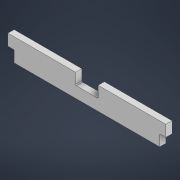
# Autodesk Inventor part: Breadth Board
Saved by Autodesk Inventor 2021 (Build 250183000, 183)
## iProperties
Created: 2021-03-26
Part Number: Breadth Board
Material: Generic
Document SubType Name: Modeling
Designer: allen
Density: 1 g/cm^3
Appearance: Default
Author: allen
Autodesk Inventor part; units mm, degrees
ref_plane "YZ Plane" through (0, 0, 0) normal (1, 0, 0) x (0, 1, 0)
ref_plane "XZ Plane" through (0, 0, 0) normal (0, 1, 0) x (-1, 0, 0)
sketch "Sketch1" plane through (0, 0, 0) normal (0, 0, 1) x (1, 0, 0)
  line L0 (0, 0) -> (384, 0)
  line L1 (384, 0) -> (384, 55)
  line L2 (384, 55) -> (0, 55)
  line L3 (0, 55) -> (0, 0)
  dimension "d0" = 55
  dimension "d1" = 384
  constraints: 8 end point, 2 parallel, 1 horizontal, 1 perpendicular
  measures "d0" distance of L2.end L0.start
  measures "d1" distance of L0.start L0.end
extrude "Extrusion1" add sketch "Sketch1" along normal blind 15
sketch "Sketch4" plane through (0, 0, 15) normal (0, 0, 1) x (1, 0, 0)
  line L0 (0, 0) -> (15, 0)
  line L1 (15, 0) -> (15, 27.5)
  line L2 (15, 27.5) -> (0, 27.5)
  line L3 (0, 27.5) -> (0, 0)
  line L4 (384, 55) -> (0, 55) projected
  line L5 (192, 55) -> (192, 39.783)
  line L6 (164.5, 55) -> (219.5, 55)
  line L7 (219.5, 55) -> (219.5, 27.5)
  line L8 (219.5, 27.5) -> (164.5, 27.5)
  line L9 (164.5, 27.5) -> (164.5, 55)
  line L10 (384, 0) -> (369, 0)
  line L11 (369, 0) -> (369, 27.5)
  line L12 (369, 27.5) -> (384, 27.5)
  line L13 (384, 27.5) -> (384, 0)
  point P0 (192, 27.5)
  dimension "d23" = 15
  dimension "d24" = 27.5
  dimension "d25" = 55
  constraints: 26 end point, 4 parallel, 4 symmetric about line, 2 horizontal, 2 midpoint, 2 perpendicular, 1 collinear, 1 point on line, 1 vertical, 1 vertical alignment
  measures "d23" distance of L1.end L2.end
  measures "d24" distance of L0.end L1.end
  measures "d25" distance of L7.end L8.end
extrude "Extrusion2" cut sketch "Sketch4" against normal through all
ref_plane "Work Plane1" through (192, 55, 15) normal (1, 0, 0) x (0, 0, -1)
fillet "Fillet1" radius 2 4 edges at (15, 27.5, 7.5) (164.5, 27.5, 7.5) (219.5, 27.5, 7.5) (369, 27.5, 7.5)
sketch "Sketch2" plane through (0, 55, 0) normal (0, 1, 0) x (1, 0, 0)
  line L0 (7.5, -7.5) -> (376.5, -7.5)
  line L1 (0, 0) -> (0, -15) projected
  line L2 (384, 0) -> (0, 0) projected
  point P0 (192, -7.5)
  point P1 (0, -7.5)
  point P2 (192, 0)
  dimension "d4" = 369
  constraints: 3 midpoint, 2 end point, 2 horizontal alignment, 1 horizontal, 1 vertical alignment
  measures "d4" distance of L0.start L0.end
sketch "Sketch3" plane through (0, 0, 0) normal (0, 0, -1) x (-1, 0, 0)
  line L0 (-384, 0) -> (-384, 55) projected
  line L1 (0, 0) -> (-384, 0) projected
  line L2 (0, 55) -> (0, 0) projected
  line L3 (-384, 55) -> (0, 55) projected
  line L4 (-7.5, 10) -> (-376.5, 10)
  line L5 (-376.5, 45) -> (-7.5, 45)
  dimension "d12" = 10
  dimension "d20" = 10
  dimension "d21" = 7.5
  dimension "d22" = 7.5
  constraints: 4 coincident, 4 end point, 2 vertical alignment
  measures "d12" distance between parallel lines of L3 L5
  measures "d20" distance between parallel lines of L1 L4
  measures "d21" distance from line of L2 point (-7.5, 45)
  measures "d22" distance from line of L0 point (-376.5, 45)
equation "\"d20\" = d12"
equation "\"d22\" = d21"
body "Solid1"
